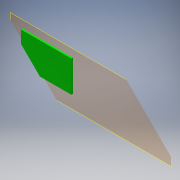
# Autodesk Inventor part: PCBQPad
Saved by Autodesk Inventor 2016 (Build 200138000, 138)
## iProperties
Created: 2018-10-10
Part Number: PCBQPad
Material: Generic
Document SubType Name: Modeling
Designer: vtolenti89
Density: 1 g/cm^3
Appearance: Default
Author: vtolenti89
Autodesk Inventor part; units mm, degrees
ref_plane "YZ Plane" through (0, 0, 0) normal (1, 0, 0) x (0, 1, 0)
ref_plane "XZ Plane" through (0, 0, 0) normal (0, 1, 0) x (-1, 0, 0)
ref_plane "XY Plane" through (0, 0, 0) normal (0, 0, 1) x (1, 0, 0)
ref_plane "Work Plane1" through (0, 0, 0) normal (0, 0, 1) x (1, 0, 0)
sketch "Sketch1" plane through (0, 0, 0) normal (0, 0, 1) x (1, 0, 0)
  line L0 (-150, 43.6) -> (-150, 12.6) construction
  line L1 (-150, 12.6) -> (-98, 12.6) construction
  line L2 (-98, 12.6) -> (-98, 43.6) construction
  line L3 (-98.2, 44.6) -> (-149.8, 44.6)
  line L4 (-149.8, 44.6) -> (-149.8, 12.6)
  line L5 (-149.8, 12.6) -> (-98.2, 12.6)
  line L6 (-98.2, 12.6) -> (-98.2, 44.6)
  line L7 (-149, 43.6) -> (-99, 43.6) construction
  point P0 (0, 0)
  dimension "d1" = 0.2
  dimension "d2" = 0.2
  dimension "d3" = 0
  dimension "d4" = 1
  constraints: 8 end point, 2 parallel, 1 horizontal, 1 perpendicular
  measures "d1" distance between parallel lines of L0 L4
  measures "d2" distance between parallel lines of L2 L6
  measures "d3" distance between parallel lines of L1 L5
  measures "d4" distance between parallel lines of L7 L3
extrude "Extrusion1" add sketch "Sketch1" along normal blind 1.6
body "Solid1"
